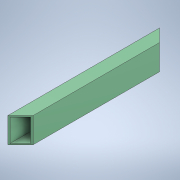
# Autodesk Inventor part: PerfilH2
Saved by Autodesk Inventor 2021 (Build 250183000, 183)
## iProperties
Created: 2021-06-11
Part Number: PerfilH2
Material: Generic
Document SubType Name: Modeling
Designer: lcper
Density: 1 g/cm^3
Appearance: Default
Author: lcper
Autodesk Inventor part; units mm, degrees
ref_plane "YZ Plane" through (0, 0, 0) normal (1, 0, 0) x (0, 1, 0)
ref_plane "XZ Plane" through (0, 0, 0) normal (0, 1, 0) x (-1, 0, 0)
ref_plane "XY Plane" through (0, 0, 0) normal (0, 0, 1) x (1, 0, 0)
sketch "Sketch1" plane through (0, 0, 0) normal (0, 0, 1) x (1, 0, 0)
  line L0 (-9.4777, 15.0257) -> (40.5223, 15.0257)
  line L1 (40.5223, 15.0257) -> (40.5223, -84.9743)
  line L2 (40.5223, -84.9743) -> (-9.4777, -84.9743)
  line L3 (-9.4777, -84.9743) -> (-9.4777, 15.0257)
  line L4 (35.5223, 10.0257) -> (-4.4777, 10.0257)
  line L5 (-4.4777, 10.0257) -> (-4.4777, -79.9743)
  line L6 (-4.4777, -79.9743) -> (35.5223, -79.9743)
  line L7 (35.5223, -79.9743) -> (35.5223, 10.0257)
  point P0 (0, 0)
  point P1 (0, 0)
  dimension "d0" = 50
  dimension "d1" = 100
  dimension "d2" = 5
  dimension "d3" = 90
  dimension "d4" = 5
  dimension "d5" = 40
  constraints: 16 end point, 4 parallel, 2 horizontal, 2 perpendicular
  measures "d0" distance of L1.end L2.end
  measures "d1" distance of L0.end L1.end
  measures "d2" distance between parallel lines of L4 L0
  measures "d3" distance of L6.end L4.start
  measures "d4" distance between parallel lines of L1 L7
  measures "d5" distance of L5.end L6.end
extrude "Extrusion1" add sketch "Sketch1" along normal blind 600
sketch "Sketch2" plane through (-9.4777, 15.0257, 0) normal (0, 1, 0) x (1, 0, 0)
  line L0 (0, 0) -> (0, -600) projected
  line L1 (0, 0) -> (51.2763, -51.2763)
  line L2 (0, 0) -> (72.5157, 0) construction
  line L3 (51.2763, -51.2763) -> (51.2763, 0)
  line L4 (45, 0) -> (45, -600) projected
  line L5 (50, 0) -> (0, 0) projected
  line L6 (51.2763, 0) -> (0, 0)
  line L7 (0, 0) -> (0, -600) projected
  line L8 (0, -600) -> (50, -550)
  line L9 (50, 0) -> (50, -600) projected
  line L10 (0, -600) -> (70.7107, -600) construction
  line L11 (50, -550) -> (50, -600)
  line L12 (50, -600) -> (0, -600)
  point P0 (9.4777, 0)
  dimension "d8" = 45
  dimension "d11" = 45
  constraints: 16 end point, 2 equal length, 2 horizontal, 2 perpendicular, 1 collinear, 1 parallel, 1 point on line
  measures "d8" angle of L1 L2
  measures "d11" angle of L10 L8
extrude "Extrusion2" cut sketch "Sketch2" against normal blind 600 contours L5 L4 L1 | L8 L4 L12 | L4 L5 L9 L1 | L8 L9 L12 L4 | L9 L6 L3 L1
body "Solid1"
